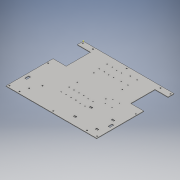
# Autodesk Inventor part: BellyPan3
Saved by Autodesk Inventor 2016 (Build 200138000, 138)
## iProperties
Created: 2017-01-26
Part Number: BellyPan3
Material: Generic
Document SubType Name: Modeling
Designer: hamblettk
Density: 1 g/cm^3
Appearance: Default
Author: hamblettk
Autodesk Inventor part; units mm, degrees
ref_plane "YZ Plane" through (0, 0, 0) normal (1, 0, 0) x (0, 1, 0)
ref_plane "XZ Plane" through (0, 0, 0) normal (0, 1, 0) x (-1, 0, 0)
ref_plane "XY Plane" through (0, 0, 0) normal (0, 0, 1) x (1, 0, 0)
sketch "Sketch1" plane through (0, 0, 0) normal (0, 1, 0) x (-1, 0, 0)
  line L0 (0, 0) -> (580.39, 0)
  line L1 (580.39, 0) -> (580.39, -495.3)
  line L2 (580.39, -495.3) -> (0, -495.3)
  line L3 (0, -495.3) -> (0, 0)
  dimension "d0" = 580.39
  dimension "d1" = 495.3
  constraints: 8 end point, 2 parallel, 1 horizontal, 1 perpendicular
  measures "d0" distance of L1.end L2.end
  measures "d1" distance of L0.end L1.end
extrude "Extrusion1" add sketch "Sketch1" along normal blind 3.175
sketch "Sketch2" plane through (0, 3.175, 0) normal (0, 1, 0) x (1, 0, 0)
  line L0 (-580.39, 0) -> (-580.39, 495.3) projected
  line L1 (-580.39, 0) -> (0, 0) projected
  line L2 (-580.39, 495.3) -> (-580.39, 0) projected
  line L3 (-580.39, 495.3) -> (0, 495.3)
  line L4 (0, 495.3) -> (-580.39, 495.3) projected
  line L5 (0, 38.1) -> (-83.82, 38.1)
  line L6 (-83.82, 38.1) -> (-83.82, 193.675)
  line L7 (-83.82, 193.675) -> (0, 193.675)
  line L8 (0, 193.675) -> (0, 38.1)
  line L9 (-580.39, 38.1) -> (-496.57, 38.1)
  line L10 (-496.57, 38.1) -> (-496.57, 193.675)
  line L11 (-496.57, 193.675) -> (-580.39, 193.675)
  line L12 (-580.39, 193.675) -> (-580.39, 38.1)
  dimension "d10" = 83.82
  dimension "d11" = 155.575
  dimension "d12" = 38.1
  dimension "d13" = 83.82
  dimension "d14" = 155.575
  dimension "d15" = 38.1
  constraints: 18 end point, 4 parallel, 2 horizontal, 2 perpendicular, 1 point on line
  measures "d10" distance of L6.end L7.end
  measures "d11" distance of L5.end L6.end
  measures "d12" distance between parallel lines of L1 L5
  measures "d13" distance of L11.end L10.end
  measures "d14" distance of L10.end L9.end
  measures "d15" distance between parallel lines of L1 L9
extrude "Extrusion2" cut sketch "Sketch2" against normal blind 3.175
sketch "Sketch3" plane through (0, 3.175, 0) normal (0, 1, 0) x (1, 0, 0)
  circle A0 centre (-9.525, 12.7) radius 3.5687
  line L0 (-580.39, 0) -> (0, 0) projected
  line L1 (0, 0) -> (0, 38.1) projected
  circle A1 centre (-9.525, 482.6) radius 3.5687
  line L2 (0, 495.3) -> (-580.39, 495.3) projected
  line L3 (0, 495.3) -> (0, 193.675) projected
  circle A2 centre (-9.525, 234.95) radius 3.5687
  line L4 (-290.195, 0) -> (-290.195, 495.3)
  circle A3 centre (-570.865, 12.7) radius 3.5687
  circle A4 centre (-570.865, 482.6) radius 3.5687
  circle A5 centre (-570.865, 234.95) radius 3.5687
  dimension "d18" = 7.1374
  dimension "d19" = 12.7
  dimension "d20" = 9.525
  dimension "d21" = 7.1374
  dimension "d22" = 12.7
  dimension "d23" = 9.525
  dimension "d24" = 7.1374
  dimension "d25" = 9.525
  dimension "d26" = 247.65
  constraints: 6 centre point, 3 symmetric about line, 2 end point, 2 midpoint, 3 other
  measures "d18" diameter of A0
  measures "d19" distance from line of L0 A0.centre
  measures "d20" distance from line of L1 A0.centre
  measures "d21" diameter of A1
  measures "d22" distance from line of L2 A1.centre
  measures "d23" distance from line of L3 A1.centre
  measures "d24" diameter of A2
  measures "d25" distance from line of L3 A2.centre
  measures "d26" distance of A1.centre A2.centre
extrude "Extrusion3" cut sketch "Sketch3" against normal blind 3.175
sketch "Sketch4" plane through (0, 3.175, 0) normal (0, 1, 0) x (1, 0, 0)
  line L0 (-29.845, 367.4364) -> (-29.845, 392.8364)
  line L1 (0, 495.3) -> (-580.39, 495.3) projected
  line L2 (0, 495.3) -> (0, 193.675) projected
  line L3 (-550.545, 367.4364) -> (-556.895, 367.4364)
  line L4 (-556.895, 367.4364) -> (-556.895, 392.8364)
  line L5 (-556.895, 392.8364) -> (-550.545, 392.8364)
  line L6 (-550.545, 392.8364) -> (-550.545, 367.4364)
  line L7 (-29.845, 392.8364) -> (-23.495, 392.8364)
  line L8 (-29.845, 367.4364) -> (-23.495, 367.4364)
  line L9 (-23.495, 367.4364) -> (-23.495, 392.8364)
  point P0 (0, 0)
  dimension "d30" = 25.4
  dimension "d33" = 6.35
  dimension "d34" = 25.4
  dimension "d35" = 102.4636
  dimension "d36" = 520.7
  dimension "d37" = 6.35
  dimension "d38" = 6.35
  constraints: 16 end point, 3 horizontal, 2 parallel, 1 perpendicular
  measures "d30" distance of L0.start L0.end
  measures "d33" distance of L4.end L5.end
  measures "d34" distance of L3.end L4.end
  measures "d35" distance between parallel lines of L1 L5
  measures "d36" distance between parallel lines of L6 L0
  measures "d37" distance of L0.end L7.end
  measures "d38" distance of L0.start L8.end
extrude "Extrusion4" cut sketch "Sketch4" against normal blind 3.175
sketch "Sketch5" plane through (0, 3.175, 0) normal (0, 1, 0) x (1, 0, 0)
  circle A0 centre (-115.57, 377.571) radius 3.5687
  line L0 (-83.82, 193.675) -> (0, 193.675) projected
  line L1 (-83.82, 38.1) -> (-83.82, 193.675) projected
  point P0 (0, 0)
  dimension "d42" = 7.1374
  dimension "d43" = 183.896
  dimension "d44" = 31.75
  constraints: 1 centre point
  measures "d42" diameter of A0
  measures "d43" distance from line of L0 A0.centre
  measures "d44" distance from line of L1 A0.centre
extrude "Extrusion5" cut sketch "Sketch5" against normal blind 3.175
sketch "Sketch6" plane through (-559.9549, 0, -0.1431) normal (0, -1, 0) x (0, 0, 1)
  circle A0 centre (-350.8851, -350.2396) radius 2.2497
  circle A1 centre (-350.9114, -319.1371) radius 2.2497
  circle A2 centre (-350.938, -287.5981) radius 2.2497
  ellipse E0 centre (-354.1933, -225.6154) end of major axis (-352.0021, -225.6135) minor radius 2.1905
  ellipse E1 centre (-354.2089, -194.5782) end of major axis (-352.0176, -194.5764) minor radius 2.1899
  ellipse E2 centre (-303.4089, -194.5392) end of major axis (-301.2176, -194.5374) minor radius 2.1899
  ellipse E3 centre (-303.3933, -225.5744) end of major axis (-301.2021, -225.5726) minor radius 2.1905
  ellipse E4 centre (-300.1641, -256.8149) end of major axis (-302.6771, -256.817) minor radius 2.5126
  circle A3 centre (-300.138, -287.5552) radius 2.513
  circle A4 centre (-300.1114, -319.0942) radius 2.513
  circle A5 centre (-300.0851, -350.1948) radius 2.513
  circle A6 centre (-350.8851, -350.2396) radius 2.513
  circle A7 centre (-350.9114, -319.1371) radius 2.413
  circle A8 centre (-350.938, -287.5981) radius 2.513
  ellipse E5 centre (-350.9641, -256.8541) end of major axis (-348.5511, -256.8521) minor radius 2.4126
  circle A9 centre (-246.6296, -350.841) radius 2.667
  circle A10 centre (-246.9059, -168.5708) radius 2.667
  circle A11 centre (-142.512, -168.4126) radius 2.667
  circle A12 centre (-142.2357, -350.6828) radius 2.667
  ellipse E6 centre (-101.9617, -356.43) end of major axis (-104.3747, -356.43) minor radius 2.413
  ellipse E7 centre (-51.1617, -356.43) end of major axis (-53.5747, -356.43) minor radius 2.413
  ellipse E8 centre (-51.1617, -323.2691) end of major axis (-53.5747, -323.2691) minor radius 2.413
  ellipse E9 centre (-101.9617, -323.2691) end of major axis (-104.3747, -323.2691) minor radius 2.413
  ellipse E10 centre (-105.1502, -292.1816) end of major axis (-107.3414, -292.1816) minor radius 2.1913
  ellipse E11 centre (-105.1502, -261.0646) end of major axis (-107.3414, -261.0646) minor radius 2.1913
  ellipse E12 centre (-54.3502, -292.1816) end of major axis (-56.5414, -292.1816) minor radius 2.1913
  ellipse E13 centre (-54.3502, -261.0646) end of major axis (-56.5414, -261.0646) minor radius 2.1913
  circle A13 centre (-42.4909, -216.236) radius 2.5
  circle A14 centre (-101.1909, -216.2459) radius 2.5
  circle A15 centre (-100.642, -173.7423) radius 2.5
  circle A16 centre (-41.942, -173.7324) radius 2.5
  circle A17 centre (-275.3803, -143.6352) radius 1.905
  circle A18 centre (-227.6284, -143.5398) radius 1.905
  circle A19 centre (-227.7168, -100.4868) radius 1.905
  circle A20 centre (-275.4663, -100.5823) radius 1.905
  ellipse E14 centre (-434.736, -472.3219) end of major axis (-438.165, -472.3219) minor radius 3.429
  ellipse E15 centre (-377.586, -444.3819) end of major axis (-374.157, -444.3819) minor radius 3.429
  circle A21 centre (-12.6998, -269.8753) radius 3.5687
  circle A22 centre (-12.6998, -498.4753) radius 3.5685
  circle A23 centre (-12.6998, -41.2753) radius 3.5687
  line L0 (-438.5985, -28.3241) -> (-448.6768, -28.3241)
  line L1 (-448.6768, -28.3241) -> (-448.6768, -35.0231)
  spline S0 degree 4 poles (-448.6768, -35.0231) (-448.6704, -35.1469) (-448.3268, -35.7898) (-448.374, -35.8834) (-448.0799, -36.4264) (-448.1726, -36.1896) (-448.2118, -36.1185) (-448.2579, -36.0024) (-448.3038, -35.9039) (-448.3418, -35.758) (-448.3871, -35.6424) (-448.4089, -35.5495) (-448.4284, -35.4842) knots 0 0 0 0 0 0.319187 0.416777 0.496886 0.564137 0.63159 0.699175 0.766403 0.833328 1 1 1 1 1
  line L2 (-448.4284, -35.4842) -> (-438.847, -35.4842)
  spline S1 degree 4 poles (-438.847, -35.4842) (-438.8355, -35.6171) (-438.8088, -35.8104) (-438.7923, -36.0459) (-438.74, -36.3561) (-438.7353, -36.5543) (-438.7189, -36.7533) (-438.7047, -36.966) (-438.6926, -37.1615) (-438.649, -37.7375) (-438.6347, -34.9543) (-438.603, -36.3425) (-438.5985, -35.0231) knots 0 0 0 0 0 0.176534 0.246794 0.316361 0.385081 0.452716 0.516863 0.592826 0.686487 1 1 1 1 1
  line L3 (-438.5985, -35.0231) -> (-438.5985, -28.3241)
  line L4 (-448.352, -20.7549) -> (-438.5985, -20.7549)
  line L5 (-448.352, -23.9299) -> (-448.352, -20.7549)
  line L6 (-438.5985, -23.9299) -> (-448.352, -23.9299)
  line L7 (-438.5985, -20.7549) -> (-438.5985, -23.9299)
  line L8 (-337.0695, -35.4845) -> (-347.0864, -35.4845)
  line L9 (-347.0864, -35.4845) -> (-347.0864, -28.3951)
  line L10 (-346.8284, -35.4842) -> (-337.247, -35.4842)
  line L11 (-337.0695, -28.3951) -> (-337.0695, -35.4845)
  ellipse E16 centre (-337.324, -28.3952) end of major axis (-337.5783, -28.3952) minor radius 0.0044 (-337.0698, -28.3951) -> (-337.3234, -28.3907) ccw
  line L12 (-346.752, -28.3907) -> (-337.3234, -28.3907)
  line L13 (-347.0768, -168.6282) -> (-336.9985, -168.6282)
  line L14 (-347.0768, -161.9292) -> (-347.0768, -168.6282)
  spline S2 degree 4 poles (-346.8284, -161.4681) (-346.8345, -161.4907) (-346.8548, -161.5224) (-346.866, -161.5641) (-346.9188, -161.6134) (-346.9239, -161.6512) (-346.9438, -161.6887) (-346.9614, -161.7268) (-346.9829, -161.7655) (-347.0152, -161.8204) (-347.0445, -161.8664) (-347.0653, -161.9032) (-347.0768, -161.9292) knots 0 0 0 0 0 0.20105 0.283621 0.36616 0.448186 0.528891 0.611653 0.69647 0.782907 1 1 1 1 1
  line L15 (-337.247, -161.4681) -> (-346.8284, -161.4681)
  spline S3 degree 4 poles (-336.9985, -161.9292) (-336.9958, -161.9015) (-336.9964, -161.863) (-337.0082, -161.8163) (-337.0309, -161.7618) (-337.0501, -161.7233) (-337.0694, -161.6844) (-337.0931, -161.647) (-337.1067, -161.6044) (-337.1672, -161.5637) (-337.1937, -161.5193) (-337.2278, -161.4909) (-337.247, -161.4681) knots 0 0 0 0 0 0.204508 0.285632 0.366887 0.448421 0.530172 0.613501 0.698079 0.783711 1 1 1 1 1
  line L16 (-336.9985, -168.6282) -> (-336.9985, -161.9292)
  line L17 (-337.0695, -176.1974) -> (-337.0695, -173.0224)
  line L18 (-346.8284, -176.1974) -> (-337.0695, -176.1974)
  line L19 (-337.0695, -173.0224) -> (-346.8284, -173.0224)
  line L20 (-346.8284, -173.0224) -> (-346.8284, -176.1974)
  line L21 (-448.6768, -168.6282) -> (-438.5985, -168.6282)
  line L22 (-438.5985, -168.6282) -> (-438.5985, -161.9292)
  line L23 (-438.847, -161.4681) -> (-448.4284, -161.4681)
  spline S4 degree 4 poles (-438.5985, -161.9292) (-438.5956, -161.9004) (-438.5959, -161.8608) (-438.608, -161.8132) (-438.6308, -161.7581) (-438.65, -161.7195) (-438.6693, -161.6806) (-438.6931, -161.6434) (-438.7067, -161.6006) (-438.767, -161.5617) (-438.7937, -161.5178) (-438.8278, -161.4904) (-438.847, -161.4681) knots 0 0 0 0 0 0.207118 0.288634 0.370017 0.451528 0.533181 0.616216 0.700347 0.785405 1 1 1 1 1
  spline S5 degree 4 poles (-448.4284, -161.4681) (-448.4341, -161.492) (-448.4548, -161.524) (-448.4648, -161.5681) (-448.5197, -161.6155) (-448.5237, -161.6553) (-448.5435, -161.6931) (-448.5609, -161.7317) (-448.5824, -161.7702) (-448.6147, -161.8241) (-448.6445, -161.8685) (-448.6655, -161.9037) (-448.6768, -161.9292) knots 0 0 0 0 0 0.203293 0.286347 0.369285 0.451683 0.532797 0.615573 0.700003 0.785679 1 1 1 1 1
  line L24 (-448.6768, -161.9292) -> (-448.6768, -168.6282)
  line L25 (-448.6768, -173.0224) -> (-448.6768, -176.1974)
  line L26 (-438.5985, -173.0224) -> (-448.6768, -173.0224)
  line L27 (-448.6768, -176.1974) -> (-438.5985, -176.1974)
  line L28 (-438.5985, -176.1974) -> (-438.5985, -173.0224)
  line L29 (-347.0864, -35.4845) -> (-337.0698, -35.4845)
  line L30 (-337.0698, -35.4845) -> (-337.0698, -28.3951)
  line L31 (-337.0698, -28.3951) -> (-347.0864, -28.3951)
  line L32 (-347.0864, -28.3951) -> (-347.0864, -35.4845)
  line L33 (-448.6768, -28.3241) -> (-438.6023, -28.3241)
  line L34 (-438.6023, -28.3241) -> (-438.6023, -35.4845)
  line L35 (-438.6023, -35.4845) -> (-448.6768, -35.4845)
  line L36 (-448.6768, -35.4845) -> (-448.6768, -28.3241)
  line L37 (-438.5985, -20.7549) -> (-448.352, -20.7549)
  line L38 (-448.352, -20.7549) -> (-448.352, -23.9299)
  line L39 (-448.352, -23.9299) -> (-438.5985, -23.9299)
  line L40 (-438.5985, -23.9299) -> (-438.5985, -20.7549)
  line L41 (-337.0698, -28.3951) -> (-347.0864, -28.3951)
  line L42 (-347.0864, -28.3951) -> (-347.0864, -35.4845)
  line L43 (-347.0864, -35.4845) -> (-337.0698, -35.4845)
  line L44 (-337.0698, -35.4845) -> (-337.0698, -28.3951)
  line L45 (-347.0864, -23.9299) -> (-337.0698, -23.9299)
  line L46 (-337.0698, -23.9299) -> (-337.0698, -20.7549)
  line L47 (-337.0698, -20.7549) -> (-347.0864, -20.7549)
  line L48 (-347.0864, -20.7549) -> (-347.0864, -23.9299)
  point P0 (0, 0)
  point P1 (-448.5054, -35.4661)
  point P2 (-448.3273, -35.8997)
  point P3 (-448.1877, -36.2205)
  point P4 (-448.1299, -36.3138)
  point P5 (-448.1658, -36.2134)
  point P6 (-448.2133, -36.1093)
  point P7 (-448.2581, -36.0052)
  point P8 (-448.3006, -35.9011)
  point P9 (-448.3332, -35.7979)
  point P10 (-448.3668, -35.6935)
  point P11 (-448.3988, -35.5889)
  point P12 (-438.8246, -35.6983)
  point P13 (-438.8008, -35.9147)
  point P14 (-438.7746, -36.1347)
  point P15 (-438.7459, -36.3584)
  point P16 (-438.7328, -36.558)
  point P17 (-438.7191, -36.7585)
  point P18 (-438.7053, -36.959)
  point P19 (-438.692, -37.1576)
  point P20 (-438.6782, -37.2828)
  point P21 (-438.6501, -36.7046)
  point P22 (-438.6207, -35.8647)
  point P23 (-346.8424, -161.5027)
  point P24 (-346.8602, -161.5386)
  point P25 (-346.8832, -161.5761)
  point P26 (-346.9133, -161.6159)
  point P27 (-346.9269, -161.6515)
  point P28 (-346.943, -161.688)
  point P29 (-346.9615, -161.7256)
  point P30 (-346.9826, -161.7643)
  point P31 (-347.0061, -161.8045)
  point P32 (-347.0314, -161.846)
  point P33 (-347.0561, -161.8881)
  point P34 (-336.9975, -161.8846)
  point P35 (-337.0033, -161.8423)
  point P36 (-337.0152, -161.8017)
  point P37 (-337.0314, -161.7622)
  point P38 (-337.05, -161.7235)
  point P39 (-337.0701, -161.6851)
  point P40 (-337.0907, -161.6468)
  point P41 (-337.1116, -161.6086)
  point P42 (-337.1475, -161.5739)
  point P43 (-337.1813, -161.5388)
  point P44 (-337.2138, -161.5034)
  point P45 (-438.5972, -161.8828)
  point P46 (-438.6031, -161.8393)
  point P47 (-438.6152, -161.7981)
  point P48 (-438.6313, -161.7584)
  point P49 (-438.65, -161.7196)
  point P50 (-438.6701, -161.6812)
  point P51 (-438.6908, -161.643)
  point P52 (-438.7117, -161.6049)
  point P53 (-438.7475, -161.5713)
  point P54 (-438.7813, -161.537)
  point P55 (-438.8138, -161.5025)
  point P56 (-448.4423, -161.5044)
  point P57 (-448.46, -161.5414)
  point P58 (-448.4831, -161.5794)
  point P59 (-448.5136, -161.6185)
  point P60 (-448.5269, -161.6553)
  point P61 (-448.5428, -161.6926)
  point P62 (-448.5612, -161.7306)
  point P63 (-448.5822, -161.7693)
  point P64 (-448.6059, -161.8087)
  point P65 (-448.6313, -161.8489)
  point P66 (-448.6562, -161.8893)
  constraints: 98 end point, 24 centre point, 10 parallel, 5 horizontal, 5 perpendicular, 1 point on line, 115 other
extrude "Extrusion6" cut sketch "Sketch6" against normal blind 25.4 contours A2 | E0 | E1 | E2 | E3 | E4 | A3 | A4 | A5 | A6 | A7 | E5 | A9 | A10 | A11 | A12 | E6 | E7 | E8 | E9 | E10 | E11 | E12 | E13 | A13 | A14 | A15 | A16 | A17 | A18 | A19 | A20 | E14 | E15 | L34 L35 L2 S0 L1 L0 | S0 L35 L36 | L4 L7 L6 L5 | L8 L9 L31 L11 | L14 S2 L15 S3 L16 L13 | L18 L20 L19 L17 | L24 S5 L23 S4 L22 L21 | L26 L28 L27 L25 | L48 L47 L46 L45
sketch "Sketch7" plane through (0, 0, 0) normal (0, -1, 0) x (1, 0, 0)
  circle A0 centre (-290.195, -12.7) radius 3.5687
  line L0 (0, 0) -> (-580.39, 0) projected
  line L1 (0, -38.1) -> (0, 0) projected
  circle A1 centre (-74.295, -12.7) radius 3.5687
  circle A2 centre (-506.095, -12.7) radius 3.5687
  circle A3 centre (-290.195, -482.6) radius 3.5687
  line L2 (-580.39, -495.3) -> (0, -495.3) projected
  line L3 (0, -495.3) -> (0, -193.675) projected
  circle A4 centre (-506.095, -482.6) radius 3.5687
  circle A5 centre (-74.295, -482.6) radius 3.5687
  dimension "d50" = 7.1374
  dimension "d51" = 12.7
  dimension "d52" = 290.195
  dimension "d53" = 7.1374
  dimension "d54" = 12.7
  dimension "d55" = 215.9
  dimension "d56" = 7.1374
  dimension "d57" = 12.7
  dimension "d58" = 215.9
  dimension "d59" = 7.1374
  dimension "d60" = 12.7
  dimension "d61" = 290.195
  dimension "d62" = 7.1374
  dimension "d63" = 215.9
  dimension "d64" = 7.1374
  dimension "d65" = 215.9
  constraints: 6 centre point
  measures "d50" diameter of A0
  measures "d51" distance from line of L0 A0.centre
  measures "d52" distance from line of L1 A0.centre
  measures "d53" diameter of A1
  measures "d54" distance from line of L0 A1.centre
  measures "d55" distance of A0.centre A1.centre
  measures "d56" diameter of A2
  measures "d57" distance from line of L0 A2.centre
  measures "d58" distance of A0.centre A2.centre
  measures "d59" diameter of A3
  measures "d60" distance from line of L2 A3.centre
  measures "d61" distance from line of L3 A3.centre
  measures "d62" diameter of A4
  measures "d63" distance of A3.centre A4.centre
  measures "d64" diameter of A5
  measures "d65" distance of A3.centre A5.centre
extrude "Extrusion7" cut sketch "Sketch7" against normal blind 3.175
sketch "Sketch8" plane through (0, 3.175, 0) normal (0, 1, 0) x (1, 0, 0)
  line L0 (-29.845, 392.8364) -> (-23.495, 392.8364) projected
  line L1 (-23.495, 392.8364) -> (-17.145, 392.8364)
  line L2 (-17.145, 392.8364) -> (-17.145, 367.4364)
  line L3 (-17.145, 367.4364) -> (-23.495, 367.4364)
  line L4 (-23.495, 367.4364) -> (-23.495, 392.8364)
  line L5 (-556.793, 392.8364) -> (-563.143, 392.8364)
  line L6 (-563.143, 392.8364) -> (-563.143, 367.4364)
  line L7 (-563.143, 367.4364) -> (-556.793, 367.4364)
  line L8 (-556.793, 367.4364) -> (-556.793, 392.8364)
  point P0 (0, 0)
  dimension "d68" = 6.35
  dimension "d69" = 25.4
  dimension "d70" = 6.35
  dimension "d71" = 25.4
  constraints: 16 end point, 4 parallel, 2 horizontal, 2 perpendicular
  measures "d68" distance of L2.end L3.end
  measures "d69" distance of L1.end L2.end
  measures "d70" distance of L7.end L6.end
  measures "d71" distance of L6.end L5.end
extrude "Extrusion8" cut sketch "Sketch8" against normal blind 3.175
fillet "Fillet1" radius 0.762 8 edges at (-17.145, 1.5875, -367.4364) (-29.845, 1.5875, -367.4364) (-29.845, 1.5875, -392.8364) (-17.145, 1.5875, -392.8364) (-550.545, 1.5875, -367.4364) (-563.143, 1.5875, -367.4364) (-563.143, 1.5875, -392.8364) (-550.545, 1.5875, -392.8364)
fillet "Fillet2" radius 0.762 28 edges at (-539.2, 1.5875, -337.2129) (-539.2, 1.5875, -347.2295) (-536.025, 1.5875, -347.2295) (-536.025, 1.5875, -337.2129) (-524.4704, 1.5875, -337.2129) (-524.4704, 1.5875, -347.2295) (-531.5598, 1.5875, -347.2295) (-531.5598, 1.5875, -337.2129) (-539.2, 1.5875, -438.7416) (-539.2, 1.5875, -448.495) (-536.025, 1.5875, -448.495) (-536.025, 1.5875, -438.7416) (-524.4704, 1.5875, -438.7453) (-531.6308, 1.5875, -448.8199) (-524.4704, 1.5875, -448.8199) (-531.6308, 1.5875, -438.7453) (-391.3268, 1.5875, -337.1416) (-391.3268, 1.5875, -347.2199) (-383.7576, 1.5875, -346.9714) (-383.7576, 1.5875, -337.2126) (-386.9326, 1.5875, -346.9714) (-386.9326, 1.5875, -337.2126) (-391.3268, 1.5875, -438.7416) (-391.3268, 1.5875, -448.8199) (-383.7576, 1.5875, -448.8199) (-383.7576, 1.5875, -438.7416) (-386.9326, 1.5875, -448.8199) (-386.9326, 1.5875, -438.7416)
sketch "Sketch9" plane through (0, 3.175, 0) normal (0, 1, 0) x (1, 0, 0)
  point P0 (0, 0)
sketch "Sketch10" plane through (0, 3.175, 0) normal (0, 1, 0) x (1, 0, 0)
  line L0 (-398.4868, 337.39) -> (-398.4868, 346.9714) projected
  line L1 (-398.0257, 347.2199) -> (-392.0888, 347.2199) projected
  spline S0 degree 5 poles (-398.4868, 346.9714) (-398.4645, 346.9775) (-398.4428, 346.9914) (-398.4206, 347) (-398.3985, 347.011) (-398.3675, 347.0351) (-398.358, 347.0439) (-398.3483, 347.0517) (-398.3382, 347.0575) (-398.3163, 347.0662) (-398.3045, 347.069) (-398.2928, 347.0731) (-398.2813, 347.079) (-398.2502, 347.0942) (-398.2305, 347.1036) (-398.2109, 347.1138) (-398.1913, 347.1251) (-398.143, 347.1534) (-398.1142, 347.1713) (-398.085, 347.1896) (-398.0554, 347.2067) (-398.0257, 347.2199) knots 0 0 0 0 0 0 0.242072 0.242072 0.242072 0.242072 0.353091 0.353091 0.353091 0.353091 0.478438 0.478438 0.478438 0.478438 0.690196 0.690196 0.690196 0.690196 1 1 1 1 1 1 projected
  spline S1 degree 5 poles (-398.0257, 337.1416) (-398.0798, 337.1363) (-398.1341, 337.1418) (-398.1809, 337.1691) (-398.2293, 337.1903) (-398.2898, 337.2243) (-398.3037, 337.2324) (-398.3184, 337.2388) (-398.3333, 337.2448) (-398.3559, 337.262) (-398.3646, 337.2711) (-398.3727, 337.281) (-398.3809, 337.2909) (-398.4085, 337.3191) (-398.4292, 337.3347) (-398.4487, 337.3528) (-398.4668, 337.3732) (-398.4868, 337.39) knots 0 0 0 0 0 0 0.499436 0.499436 0.499436 0.499436 0.649824 0.649824 0.649824 0.649824 0.7612 0.7612 0.7612 0.7612 1 1 1 1 1 1 projected
  line L2 (-392.0888, 337.1416) -> (-398.0257, 337.1416) projected
  arc A0 (-392.0888, 337.1416) -> (-391.3268, 337.9036) centre (-392.0888, 337.9036) ccw projected
  line L3 (-391.3268, 346.4579) -> (-391.3268, 337.9036) projected
  arc A1 (-391.3268, 346.4579) -> (-392.0888, 347.2199) centre (-392.0888, 346.4579) ccw projected
  line L4 (-391.3268, 448.0579) -> (-391.3268, 439.5036) projected
  line L5 (-392.0888, 438.7416) -> (-398.0257, 438.7416) projected
  line L6 (-398.4868, 438.99) -> (-398.4868, 448.5714) projected
  spline S2 degree 5 poles (-398.0257, 438.7416) (-398.0812, 438.736) (-398.1365, 438.741) (-398.1836, 438.7687) (-398.2325, 438.7898) (-398.2932, 438.8241) (-398.3072, 438.8323) (-398.322, 438.8388) (-398.3372, 438.8447) (-398.3594, 438.862) (-398.3677, 438.871) (-398.3755, 438.8809) (-398.3834, 438.8906) (-398.4101, 438.9188) (-398.4305, 438.9345) (-398.4496, 438.9526) (-398.4672, 438.9731) (-398.4868, 438.99) knots 0 0 0 0 0 0 0.502139 0.502139 0.502139 0.502139 0.653481 0.653481 0.653481 0.653481 0.762608 0.762608 0.762608 0.762608 1 1 1 1 1 1 projected
  arc A2 (-392.0888, 438.7416) -> (-391.3268, 439.5036) centre (-392.0888, 439.5036) ccw projected
  line L7 (-398.0257, 448.8199) -> (-392.0888, 448.8199) projected
  spline S3 degree 4 poles (-398.4868, 448.5714) (-398.4604, 448.5777) (-398.4357, 448.5947) (-398.4091, 448.6026) (-398.3704, 448.6293) (-398.3572, 448.6426) (-398.3434, 448.6541) (-398.3104, 448.6683) (-398.291, 448.6701) (-398.2731, 448.6806) (-398.2232, 448.7047) (-398.1914, 448.7203) (-398.1603, 448.7399) (-398.1036, 448.7759) (-398.0781, 448.7928) (-398.0522, 448.8082) (-398.0257, 448.8199) knots 0 0 0 0 0 0.221377 0.221377 0.221377 0.348729 0.348729 0.348729 0.50517 0.50517 0.50517 0.777595 0.777595 0.777595 1 1 1 1 1 projected
  arc A3 (-391.3268, 448.0579) -> (-392.0888, 448.8199) centre (-392.0888, 448.0579) ccw projected
  point P0 (0, 0)
  constraints: 4 other
extrude "Extrusion9" add sketch "Sketch10" against normal blind 3.175
sketch "Sketch11" plane through (0, 3.175, 0) normal (0, 1, 0) x (1, 0, 0)
  line L0 (-384.5196, 337.2126) -> (-386.1706, 337.2126) projected
  line L1 (-386.1706, 346.9714) -> (-384.5196, 346.9714) projected
  line L2 (-392.0888, 337.2126) -> (-397.7276, 337.2126)
  line L3 (-398.4896, 337.9746) -> (-398.4896, 346.2042)
  line L4 (-397.7276, 346.9662) -> (-392.0888, 346.9662)
  line L5 (-391.3268, 346.2042) -> (-391.3268, 337.9746)
  line L6 (-386.9326, 337.9746) -> (-386.9326, 346.2094) projected
  line L7 (-386.1706, 448.8199) -> (-384.5196, 448.8199) projected
  line L8 (-384.5196, 438.7416) -> (-386.1706, 438.7416) projected
  line L9 (-392.0888, 438.7416) -> (-397.7276, 438.7416)
  line L10 (-398.4896, 439.5036) -> (-398.4896, 448.0579)
  line L11 (-397.7276, 448.8199) -> (-392.0888, 448.8199)
  line L12 (-391.3268, 448.0579) -> (-391.3268, 439.5036)
  line L13 (-386.9326, 448.0579) -> (-386.9326, 439.5036) projected
  arc A0 (-398.4896, 337.9746) -> (-397.7276, 337.2126) centre (-397.7276, 337.9746) ccw
  arc A1 (-397.7276, 346.9662) -> (-398.4896, 346.2042) centre (-397.7276, 346.2042) ccw
  arc A2 (-391.3268, 346.2042) -> (-392.0888, 346.9662) centre (-392.0888, 346.2042) ccw
  arc A3 (-392.0888, 337.2126) -> (-391.3268, 337.9746) centre (-392.0888, 337.9746) ccw
  arc A4 (-392.0888, 438.7416) -> (-391.3268, 439.5036) centre (-392.0888, 439.5036) ccw
  arc A5 (-398.4896, 439.5036) -> (-397.7276, 438.7416) centre (-397.7276, 439.5036) ccw
  arc A6 (-397.7276, 448.8199) -> (-398.4896, 448.0579) centre (-397.7276, 448.0579) ccw
  arc A7 (-391.3268, 448.0579) -> (-392.0888, 448.8199) centre (-392.0888, 448.0579) ccw
  point P0 (0, 0)
  point P1 (-398.4896, 346.9662)
  point P2 (-398.4896, 337.2126)
  point P3 (-391.3268, 346.9662)
  point P4 (-398.4896, 448.8199)
  point P5 (-391.3268, 448.8199)
  dimension "d78" = 7.1628
  dimension "d79" = 9.7536
  dimension "d80" = 4.3942
  dimension "d81" = 7.1628
  dimension "d82" = 4.3942
  dimension "d83" = 0.762
  constraints: 16 end point, 16 point on circle, 16 tangent, 10 point on line, 8 centre point, 7 equal radius, 4 parallel, 2 horizontal, 2 perpendicular
  measures "d78" distance of point (-398.49, 346.966) point (-391.327, 346.966)
  measures "d79" distance of point (-398.49, 337.213) point (-398.49, 346.966)
  measures "d80" distance between parallel lines of L6 L5
  measures "d81" distance of point (-398.49, 448.82) point (-391.327, 448.82)
  measures "d82" distance between parallel lines of L13 L12
  measures "d83" radius of A0
extrude "Extrusion10" cut sketch "Sketch11" against normal blind 3.175
body "Solid1"
